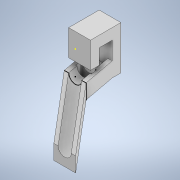
# Autodesk Inventor part: entry_ramp
Saved by Autodesk Inventor 2021 (Build 250183000, 183)
## iProperties
Created: 2021-04-02
Part Number: entry_ramp
Material: Generic
Document SubType Name: Modeling
Designer: Jawal
Density: 1 g/cm^3
Appearance: Default
Author: Jawal
Autodesk Inventor part; units mm, degrees
note: some values were not read from the file. Chosen so that the rebuilt part matches the saved one: direction of "Emboss1".
sketch "Sketch1" plane through (0, 0, 0) normal (0, 0, 1) x (1, 0, 0)
  line L0 (-12.5, 12.5) -> (12.5, 12.5)
  line L1 (12.5, 12.5) -> (12.5, -37.5)
  line L2 (12.5, -37.5) -> (-12.5, -37.5)
  line L3 (-12.5, -37.5) -> (-12.5, 12.5)
  point P0 (0, 0)
  dimension "d0" = 25
  dimension "d1" = 50
  dimension "d2" = 12.5
  dimension "d3" = 12.5
  constraints: 8 end point, 2 parallel, 1 horizontal, 1 perpendicular
  measures "d0" distance of L0.start L0.end
  measures "d1" distance of L0.end L1.end
  measures "d2" distance from line of L1 point (0, 0)
  measures "d3" distance from line of point (0, 0) L0
sketch "Sketch1 outline for Extrusion1" plane through (0, 0, 0) normal (0, 0, 1) x (1, 0, 0)
  line L0 (-12.5, 12.5) -> (-12.5, -37.5)
  line L1 (12.5, 12.5) -> (-12.5, 12.5)
  line L2 (12.5, -37.5) -> (12.5, 12.5)
  line L3 (-12.5, -37.5) -> (12.5, -37.5)
extrude "Extrusion1" add sketch "Sketch1 outline for Extrusion1" along normal blind 10
sketch "Sketch2" plane through (0, 0, 0) normal (0, 0, -1) x (-1, 0, 0)
  circle A0 centre (0, -33) radius 1.5
  circle A1 centre (0, 0) radius 7.5
  dimension "d7" = 3
  dimension "d8" = 33
  dimension "d17" = 15
  constraints: 2 centre point, 1 coincident
  measures "d7" diameter of A0
  measures "d8" distance of A0.centre point (0, 0)
  measures "d17" diameter of A1
sketch "Sketch2 outline for Extrusion2" plane through (0, 0, 0) normal (0, 0, -1) x (-1, 0, 0)
  circle A0 centre (0, -33) radius 1.5
extrude "Extrusion2" add sketch "Sketch2 outline for Extrusion2" along normal blind 6
sketch "Sketch3" plane through (0, 0, 10) normal (0, 0, 1) x (1, 0, 0)
  arc A0 (7.5, 0) -> (-7.5, 0) centre (0, 0) ccw
  line L0 (-7.5, 0) -> (-12.5, 0)
  line L1 (-12.5, 12.5) -> (-12.5, -37.5) projected
  line L2 (-12.5, 0) -> (-12.5, 12.5)
  line L3 (12.5, 12.5) -> (-12.5, 12.5) projected
  line L4 (12.5, 12.5) -> (12.5, 0)
  line L5 (12.5, -37.5) -> (12.5, 12.5) projected
  line L6 (7.5, 0) -> (12.5, 0)
  dimension "d11" = 15
  constraints: 8 end point, 2 point on circle, 2 point on line, 1 centre point, 1 coincident, 1 collinear, 1 horizontal, 1 perpendicular
  measures "d11" diameter of A0
sketch "Sketch3 outline for Extrusion3" plane through (0, 0, 10) normal (0, 0, 1) x (1, 0, 0)
  arc A0 (-7.5, 0) -> (7.5, 0) centre (0, 0) cw
  line L0 (-12.5, 0) -> (-7.5, 0)
  line L1 (-12.5, 12.5) -> (-12.5, 0)
  line L2 (12.5, 12.5) -> (-12.5, 12.5)
  line L3 (12.5, 0) -> (12.5, 12.5)
  line L4 (7.5, 0) -> (12.5, 0)
extrude "Extrusion3" add sketch "Sketch3 outline for Extrusion3" along normal blind 15
sketch "Sketch4" plane through (0, 0, 25) normal (0, 0, 1) x (1, 0, 0)
  line L0 (-12.5, 12.5) -> (-12.5, 0) projected
  line L1 (-12.5, 12.5) -> (12.5, 12.5)
  line L2 (12.5, 12.5) -> (12.5, -17.5)
  line L3 (12.5, -17.5) -> (-12.5, -17.5)
  line L4 (-12.5, -17.5) -> (-12.5, 12.5)
  point P0 (0, 0)
  dimension "d14" = 25
  dimension "d21" = 30
  constraints: 8 end point, 2 parallel, 1 horizontal, 1 perpendicular
  measures "d14" distance of L2.end L3.end
  measures "d21" distance of L1.end L2.end
sketch "Sketch4 outline for Extrusion4" plane through (0, 0, 25) normal (0, 0, 1) x (1, 0, 0)
  line L0 (-12.5, -17.5) -> (12.5, -17.5)
  line L1 (-12.5, 0) -> (-12.5, -17.5)
  line L2 (-12.5, 12.5) -> (-12.5, 0)
  line L3 (12.5, 12.5) -> (-12.5, 12.5)
  line L4 (12.5, -17.5) -> (12.5, 12.5)
extrude "Extrusion4" add sketch "Sketch4 outline for Extrusion4" along normal blind 10
sketch "Sketch5" plane through (0, 0, 0) normal (0, 0, -1) x (-1, 0, 0)
  circle A0 centre (0, 0) radius 7.5
  dimension "d18" = 15
  constraints: 1 centre point, 1 coincident
  measures "d18" diameter of A0
sketch "Sketch5 outline for Extrusion5" plane through (0, 0, 0) normal (0, 0, -1) x (-1, 0, 0)
  circle A0 centre (0, 0) radius 7.5
extrude "Extrusion5" cut sketch "Sketch5 outline for Extrusion5" against normal blind 10
sketch "Sketch6" plane through (0, 0, 10) normal (0, 0, 1) x (1, 0, 0)
  line L0 (-12.5, -20.5) -> (-12.5, -37.5)
  line L1 (-12.5, -37.5) -> (12.5, -37.5) projected
  line L2 (-12.5, -37.5) -> (12.5, -37.5)
  line L3 (12.5, -37.5) -> (12.5, -20.5)
  line L4 (12.5, -37.5) -> (12.5, 0) projected
  arc A0 (-7.5, -20.5) -> (7.5, -20.5) centre (0, -20.5) ccw
  line L5 (-12.5, -20.5) -> (-7.5, -20.5)
  line L6 (7.5, -20.5) -> (12.5, -20.5)
  line L7 (-12.5, 0) -> (-12.5, -37.5) projected
  line L8 (-12.5, -29) -> (12.5, -29)
  point P0 (0, 0)
  dimension "d22" = 15
  dimension "d23" = 17
  dimension "d24" = 17
  constraints: 12 end point, 3 point on line, 2 horizontal, 2 point on circle, 1 centre point, 1 collinear, 1 perpendicular
  measures "d22" diameter of A0
  measures "d23" distance of L1.end L3.end
  measures "d24" distance of L0.start L0.end
ref_plane "Work Plane1" through (0, -37.5, 0) normal (-1, 0, 0) x (0, 0, 1)
sketch "Sketch8" plane through (0, -37.5, 0) normal (-1, 0, 0) x (0, 0, 1)
  line L0 (10, 0) -> (10, 37.5)
  line L1 (10, 8.5) -> (40, 1.573954)
  line L2 (10, 8.5) -> (40.789123, 8.5) construction
  line L3 (0, 0) -> (10, 0)
  point P0 (0, 37.5)
  dimension "d26" = 13
  dimension "d27" = 8.5
  dimension "d32" = 30
  constraints: 4 end point, 1 equal length, 1 horizontal, 1 point on line
  measures "d26" angle of L1 L2
  measures "d27" distance between parallel lines of L3 L2
  measures "d32" distance from line of L1.end L0
sketch "Sketch6 outline for Sweep1" plane through (0, 0, 10) normal (0, 0, 1) x (1, 0, 0)
  arc A0 (7.5, -20.5) -> (-7.5, -20.5) centre (0, -20.5) cw
  line L0 (12.5, -20.5) -> (7.5, -20.5)
  line L1 (12.5, -37.5) -> (12.5, -20.5)
  line L2 (-12.5, -37.5) -> (12.5, -37.5)
  line L3 (-12.5, -20.5) -> (-12.5, -37.5)
  line L4 (-7.5, -20.5) -> (-12.5, -20.5)
sweep "Sweep1" add profiles "Sketch6 outline for Sweep1" path "Sketch8" path curves L1
thread "Thread1"
sketch "Sketch9" plane through (-12.5, -44.426046, 40) normal (0, 0, 1) x (1, 0, 0)
  point P0 (12.5, 44.426046)
sketch "Sketch10" plane through (-12.5, -44.426046, 40) normal (0, 0, 1) x (1, 0, 0)
  point P0 (12.5, 44.426046)
ref_plane "Work Plane2" through (12.5, -44.426046, 40) normal (0, -1, 0) x (1, 0, 0)
sketch "Sketch12" plane through (12.5, -44.426046, 40) normal (0, -1, 0) x (1, 0, 0)
  line L0 (-3.5, -15.5) -> (-21.5, -15.5)
  line L1 (-21.5, -15.5) -> (-21.5, -9.5)
  line L2 (-21.5, -9.5) -> (-3.5, -9.5)
  line L3 (-3.5, -9.5) -> (-3.5, -15.5)
  line L4 (0, -30) -> (0, 0) projected
  point P0 (-12.5, -40)
  dimension "d33" = 18
  dimension "d34" = 6
  dimension "d35" = 3.5
  dimension "d36" = 14.5
  constraints: 8 end point, 1 horizontal, 1 parallel, 1 perpendicular
  measures "d33" distance of L1.end L2.end
  measures "d34" distance of L0.end L1.end
  measures "d35" distance between parallel lines of L4 L3
  measures "d36" distance from line of L4.start L0
sketch "Sketch12 outline for Extrusion6" plane through (12.5, -44.426046, 40) normal (0, -1, 0) x (1, 0, 0)
  line L0 (-3.5, -15.5) -> (-3.5, -9.5)
  line L1 (-21.5, -15.5) -> (-3.5, -15.5)
  line L2 (-21.5, -9.5) -> (-21.5, -15.5)
  line L3 (-3.5, -9.5) -> (-21.5, -9.5)
extrude "Extrusion6" cut sketch "Sketch12 outline for Extrusion6" against normal blind 25
sketch "Sketch13" plane through (-12.5, -44.426046, 40) normal (0, 0, 1) x (1, 0, 0)
  line L0 (5, 17) -> (0, 17) projected
  line L1 (5, 17) -> (0, 17)
  line L2 (0, 17) -> (0, 0) projected
  line L3 (0, 17) -> (0, 0)
  line L4 (0, 0) -> (25, 0) projected
  line L5 (0, 0) -> (25, 0)
  line L6 (25, 0) -> (25, 17) projected
  line L7 (25, 0) -> (25, 17)
  arc A0 (5, 17) -> (20, 17) centre (12.5, 17) ccw projected
  line L8 (25, 17) -> (20, 17)
  arc A1 (5, 17) -> (20, 17) centre (12.5, 17) ccw
  point P0 (12.5, 44.426046)
  constraints: 10 end point, 2 collinear, 2 perpendicular, 2 point on circle, 1 centre point, 1 concentric, 1 horizontal
ref_plane "Work Plane3" through (-12.5, -44.426046, 80) normal (0, 0, 1) x (1, 0, 0)
sketch "Sketch14" plane through (-12.5, -44.426046, 80) normal (0, 0, 1) x (1, 0, 0)
  line L0 (28, -21.574) -> (28, -38.574)
  line L1 (28, -38.574) -> (53, -38.574)
  line L2 (53, -38.574) -> (53, -21.574)
  line L3 (53, -21.574) -> (48, -21.574)
  line L4 (28, -21.574) -> (33, -21.574)
  arc A0 (33, -21.574) -> (48, -21.574) centre (40.5, -21.574) ccw
  line L5 (5, 17) -> (0, 17) projected
  point P0 (12.5, 44.426046)
  dimension "d40" = 17
  dimension "d41" = 25
  dimension "d42" = 5
  dimension "d43" = 5
  dimension "d45" = 15
  dimension "d46" = 38.574
  dimension "d47" = 28
  constraints: 10 end point, 3 perpendicular, 2 point on circle, 1 centre point, 1 horizontal, 1 vertical
  measures "d40" distance of L0.start L0.end
  measures "d41" distance of L0.end L1.end
  measures "d42" distance of L2.end L3.end
  measures "d43" distance of L0.start L4.end
  measures "d45" diameter of A0
  measures "d46" distance between parallel lines of L4 L5
  measures "d47" horizontal distance of L0.start L5.end
sketch "Sketch14 outline for Loft1" plane through (-12.5, -44.426046, 80) normal (0, 0, 1) x (1, 0, 0)
  line L0 (33, -21.574) -> (28, -21.574)
  arc A0 (48, -21.574) -> (33, -21.574) centre (40.5, -21.574) cw
  line L1 (53, -21.574) -> (48, -21.574)
  line L2 (53, -38.574) -> (53, -21.574)
  line L3 (28, -38.574) -> (53, -38.574)
  line L4 (28, -21.574) -> (28, -38.574)
loft "Loft1" add profiles "Sketch14 outline for Loft1" section 1 edges at (-10, -27.426046, 40) (-12.5, -35.926046, 40) (0, -44.426046, 40) (12.5, -35.926046, 40) (10, -27.426046, 40) (0, -34.926046, 40)
sketch "Sketch15" plane through (-12.5, -37.5, 0) normal (-1, 0, 0) x (0, 0, 1)
  line L0 (6.091781, 45.785955) -> (39.829507, 45.785955) construction
  line L1 (39.829507, 45.785955) -> (39.829507, 34.540045) construction
  line L2 (39.829507, 34.540045) -> (6.091781, 34.540045) construction
  line L3 (6.091781, 34.540045) -> (6.091781, 45.785955) construction
  line L4 (6.400533, 42.737955) -> (6.400533, 45.785955)
  line L5 (6.400533, 45.785955) -> (8.307386, 45.785955)
  line L6 (8.307386, 45.785955) -> (8.307386, 45.425332)
  line L7 (8.307386, 45.425332) -> (6.805616, 45.425332)
  line L8 (6.805616, 45.425332) -> (6.805616, 44.590467)
  line L9 (6.805616, 44.590467) -> (8.206115, 44.590467)
  line L10 (8.206115, 44.590467) -> (8.206115, 44.229844)
  line L11 (8.206115, 44.229844) -> (6.805616, 44.229844)
  line L12 (6.805616, 44.229844) -> (6.805616, 43.098577)
  line L13 (6.805616, 43.098577) -> (8.307386, 43.098577)
  line L14 (8.307386, 43.098577) -> (8.307386, 42.737955)
  line L15 (8.307386, 42.737955) -> (6.400533, 42.737955)
  line L16 (10.51805, 42.737955) -> (10.132728, 42.737955)
  line L17 (10.132728, 42.737955) -> (10.132728, 44.042123)
  spline S0 degree 2 poles (10.132728, 44.042123) (10.132728, 44.200204) (10.103087, 44.471906) (10.058627, 44.553417) knots 0 0 0 1 2 2 2
  spline S1 degree 2 poles (10.058627, 44.553417) (10.011697, 44.639867) (9.843736, 44.723848) (9.700475, 44.723848) knots 0 0 0 1 2 2 2
  spline S2 degree 2 poles (9.700475, 44.723848) (9.557214, 44.723848) (9.253402, 44.570707) (9.107671, 44.447206) knots 0 0 0 1 2 2 2
  line L18 (9.107671, 44.447206) -> (9.107671, 42.737955)
  line L19 (9.107671, 42.737955) -> (8.722348, 42.737955)
  line L20 (8.722348, 42.737955) -> (8.722348, 45.02519)
  line L21 (8.722348, 45.02519) -> (9.107671, 45.02519)
  line L22 (9.107671, 45.02519) -> (9.107671, 44.770778)
  spline S3 degree 2 poles (9.107671, 44.770778) (9.280572, 44.926389) (9.614024, 45.08941) (9.801745, 45.08941) knots 0 0 0 1 2 2 2
  spline S4 degree 2 poles (9.801745, 45.08941) (10.137668, 45.08941) (10.51805, 44.644807) (10.51805, 44.222434) knots 0 0 0 1 2 2 2
  line L23 (10.51805, 44.222434) -> (10.51805, 42.737955)
  spline S5 degree 2 poles (11.750588, 42.693494) (11.436896, 42.693494) (11.083684, 43.051647) (11.083684, 43.439439) knots 0 0 0 1 2 2 2
  line L24 (11.083684, 43.439439) -> (11.083684, 44.706558)
  line L25 (11.083684, 44.706558) -> (10.824332, 44.706558)
  line L26 (10.824332, 44.706558) -> (10.824332, 45.02519)
  line L27 (10.824332, 45.02519) -> (11.083684, 45.02519)
  line L28 (11.083684, 45.02519) -> (11.083684, 45.682214)
  line L29 (11.083684, 45.682214) -> (11.469006, 45.682214)
  line L30 (11.469006, 45.682214) -> (11.469006, 45.02519)
  line L31 (11.469006, 45.02519) -> (12.177901, 45.02519)
  line L32 (12.177901, 45.02519) -> (12.177901, 44.706558)
  line L33 (12.177901, 44.706558) -> (11.469006, 44.706558)
  line L34 (11.469006, 44.706558) -> (11.469006, 43.61728)
  spline S6 degree 2 poles (11.469006, 43.61728) (11.469006, 43.444379) (11.481356, 43.254188) (11.523347, 43.172678) knots 0 0 0 1 2 2 2
  spline S7 degree 2 poles (11.523347, 43.172678) (11.557927, 43.101047) (11.713538, 43.029417) (11.846919, 43.029417) knots 0 0 0 1 2 2 2
  spline S8 degree 2 poles (11.846919, 43.029417) (11.940779, 43.029417) (12.116151, 43.086227) (12.155671, 43.103517) knots 0 0 0 1 2 2 2
  line L35 (12.155671, 43.103517) -> (12.177901, 43.103517)
  line L36 (12.177901, 43.103517) -> (12.177901, 42.757715)
  spline S9 degree 2 poles (12.177901, 42.757715) (12.06922, 42.728075) (11.846919, 42.693494) (11.750588, 42.693494) knots 0 0 0 1 2 2 2
  line L37 (13.674731, 44.612697) -> (13.654971, 44.612697)
  spline S10 degree 2 poles (13.654971, 44.612697) (13.61051, 44.625047) (13.51418, 44.629987) (13.447489, 44.629987) knots 0 0 0 1 2 2 2
  spline S11 degree 2 poles (13.447489, 44.629987) (13.291878, 44.629987) (12.985596, 44.494136) (12.847275, 44.360755) knots 0 0 0 1 2 2 2
  line L38 (12.847275, 44.360755) -> (12.847275, 42.737955)
  line L39 (12.847275, 42.737955) -> (12.461953, 42.737955)
  line L40 (12.461953, 42.737955) -> (12.461953, 45.02519)
  line L41 (12.461953, 45.02519) -> (12.847275, 45.02519)
  line L42 (12.847275, 45.02519) -> (12.847275, 44.684327)
  spline S12 degree 2 poles (12.847275, 44.684327) (13.057227, 44.872049) (13.370919, 45.02519) (13.51912, 45.02519) knots 0 0 0 1 2 2 2
  spline S13 degree 2 poles (13.51912, 45.02519) (13.5784, 45.02519) (13.637681, 45.02025) (13.674731, 45.01284) knots 0 0 0 1 2 2 2
  line L43 (13.674731, 45.01284) -> (13.674731, 44.612697)
  line L44 (15.769305, 45.02519) -> (14.539237, 41.895679)
  line L45 (14.539237, 41.895679) -> (14.126744, 41.895679)
  line L46 (14.126744, 41.895679) -> (14.536767, 42.849105)
  line L47 (14.536767, 42.849105) -> (13.706841, 45.02519)
  line L48 (13.706841, 45.02519) -> (14.121804, 45.02519)
  line L49 (14.121804, 45.02519) -> (14.746718, 43.330759)
  line L50 (14.746718, 43.330759) -> (15.369162, 45.02519)
  line L51 (15.369162, 45.02519) -> (15.769305, 45.02519)
  line L52 (19.758381, 42.737955) -> (19.232267, 42.737955)
  line L53 (19.232267, 42.737955) -> (18.268961, 43.950733)
  line L54 (18.268961, 43.950733) -> (17.804598, 43.950733)
  line L55 (17.804598, 43.950733) -> (17.804598, 42.737955)
  line L56 (17.804598, 42.737955) -> (17.399515, 42.737955)
  line L57 (17.399515, 42.737955) -> (17.399515, 45.785955)
  line L58 (17.399515, 45.785955) -> (18.184981, 45.785955)
  spline S14 degree 2 poles (18.184981, 45.785955) (18.446802, 45.785955) (18.800015, 45.729144) (18.960566, 45.625404) knots 0 0 0 1 2 2 2
  spline S15 degree 2 poles (18.960566, 45.625404) (19.121117, 45.521663) (19.306368, 45.198091) (19.306368, 44.958499) knots 0 0 0 1 2 2 2
  spline S16 degree 2 poles (19.306368, 44.958499) (19.306368, 44.625047) (18.965506, 44.173034) (18.674044, 44.064353) knots 0 0 0 1 2 2 2
  line L59 (18.674044, 44.064353) -> (19.758381, 42.737955)
  spline S17 degree 2 poles (18.883995, 44.926389) (18.883995, 45.05977) (18.790135, 45.264781) (18.691334, 45.331472) knots 0 0 0 1 2 2 2
  spline S18 degree 2 poles (18.691334, 45.331472) (18.604883, 45.388282) (18.375172, 45.435212) (18.207211, 45.435212) knots 0 0 0 1 2 2 2
  line L60 (18.207211, 45.435212) -> (17.804598, 45.435212)
  line L61 (17.804598, 45.435212) -> (17.804598, 44.289125)
  line L62 (17.804598, 44.289125) -> (18.16028, 44.289125)
  spline S19 degree 2 poles (18.16028, 44.289125) (18.335652, 44.289125) (18.614763, 44.350875) (18.711094, 44.447206) knots 0 0 0 1 2 2 2
  spline S20 degree 2 poles (18.711094, 44.447206) (18.800015, 44.531186) (18.883995, 44.768308) (18.883995, 44.926389) knots 0 0 0 1 2 2 2
  spline S21 degree 2 poles (21.245331, 42.980016) (21.1984, 42.945436) (21.040319, 42.821935) (20.966219, 42.784885) knots 0 0 0 1 2 2 2
  spline S22 degree 2 poles (20.966219, 42.784885) (20.864948, 42.730545) (20.674757, 42.673734) (20.501856, 42.673734) knots 0 0 0 1 2 2 2
  spline S23 degree 2 poles (20.501856, 42.673734) (20.361065, 42.673734) (20.106653, 42.779945) (20.010323, 42.876276) knots 0 0 0 1 2 2 2
  spline S24 degree 2 poles (20.010323, 42.876276) (19.918932, 42.970136) (19.807781, 43.246778) (19.807781, 43.399919) knots 0 0 0 1 2 2 2
  spline S25 degree 2 poles (19.807781, 43.399919) (19.807781, 43.637041) (20.007853, 43.972963) (20.225214, 44.069293) knots 0 0 0 1 2 2 2
  spline S26 degree 2 poles (20.225214, 44.069293) (20.417875, 44.158214) (20.941519, 44.224904) (21.245331, 44.242195) knots 0 0 0 1 2 2 2
  line L63 (21.245331, 44.242195) -> (21.245331, 44.316295)
  spline S27 degree 2 poles (21.245331, 44.316295) (21.245331, 44.449676) (21.16382, 44.615167) (21.08972, 44.662097) knots 0 0 0 1 2 2 2
  spline S28 degree 2 poles (21.08972, 44.662097) (21.015619, 44.709028) (20.803198, 44.738668) (20.689577, 44.738668) knots 0 0 0 1 2 2 2
  spline S29 degree 2 poles (20.689577, 44.738668) (20.556196, 44.738668) (20.195574, 44.659627) (20.015263, 44.583057) knots 0 0 0 1 2 2 2
  line L64 (20.015263, 44.583057) -> (19.993032, 44.583057)
  line L65 (19.993032, 44.583057) -> (19.993032, 44.975789)
  spline S30 degree 2 poles (19.993032, 44.975789) (20.099243, 45.00543) (20.496916, 45.07953) (20.692047, 45.07953) knots 0 0 0 1 2 2 2
  spline S31 degree 2 poles (20.692047, 45.07953) (20.929169, 45.07953) (21.252741, 45.00543) (21.381182, 44.909099) knots 0 0 0 1 2 2 2
  spline S32 degree 2 poles (21.381182, 44.909099) (21.507152, 44.815238) (21.630653, 44.516366) (21.630653, 44.301475) knots 0 0 0 1 2 2 2
  line L66 (21.630653, 44.301475) -> (21.630653, 42.737955)
  line L67 (21.630653, 42.737955) -> (21.245331, 42.737955)
  line L68 (21.245331, 42.737955) -> (21.245331, 42.980016)
  line L69 (21.245331, 43.301118) -> (21.245331, 43.935913)
  spline S33 degree 2 poles (21.245331, 43.935913) (21.10701, 43.923562) (20.689577, 43.881572) (20.558666, 43.842052) knots 0 0 0 1 2 2 2
  spline S34 degree 2 poles (20.558666, 43.842052) (20.405525, 43.795122) (20.205454, 43.59999) (20.205454, 43.427089) knots 0 0 0 1 2 2 2
  spline S35 degree 2 poles (20.205454, 43.427089) (20.205454, 43.229488) (20.427755, 43.029417) (20.640177, 43.029417) knots 0 0 0 1 2 2 2
  spline S36 degree 2 poles (20.640177, 43.029417) (20.820488, 43.029417) (21.11689, 43.185028) (21.245331, 43.301118) knots 0 0 0 1 2 2 2
  line L70 (24.765104, 42.737955) -> (24.765104, 44.061883)
  spline S37 degree 2 poles (24.765104, 44.061883) (24.765104, 44.219964) (24.740404, 44.489196) (24.700883, 44.563297) knots 0 0 0 1 2 2 2
  spline S38 degree 2 poles (24.700883, 44.563297) (24.661363, 44.644807) (24.510692, 44.723848) (24.379781, 44.723848) knots 0 0 0 1 2 2 2
  spline S39 degree 2 poles (24.379781, 44.723848) (24.26122, 44.723848) (23.989519, 44.578117) (23.846258, 44.439796) knots 0 0 0 1 2 2 2
  spline S40 degree 2 poles (23.846258, 44.439796) (23.848728, 44.405216) (23.853668, 44.308885) (23.853668, 44.244665) knots 0 0 0 1 2 2 2
  line L71 (23.853668, 44.244665) -> (23.853668, 42.737955)
  line L72 (23.853668, 42.737955) -> (23.468345, 42.737955)
  line L73 (23.468345, 42.737955) -> (23.468345, 44.061883)
  spline S41 degree 2 poles (23.468345, 44.061883) (23.468345, 44.219964) (23.443645, 44.489196) (23.404125, 44.563297) knots 0 0 0 1 2 2 2
  spline S42 degree 2 poles (23.404125, 44.563297) (23.364605, 44.644807) (23.213934, 44.723848) (23.083023, 44.723848) knots 0 0 0 1 2 2 2
  spline S43 degree 2 poles (23.083023, 44.723848) (22.959522, 44.723848) (22.68535, 44.568237) (22.556909, 44.447206) knots 0 0 0 1 2 2 2
  line L74 (22.556909, 44.447206) -> (22.556909, 42.737955)
  line L75 (22.556909, 42.737955) -> (22.171587, 42.737955)
  line L76 (22.171587, 42.737955) -> (22.171587, 45.02519)
  line L77 (22.171587, 45.02519) -> (22.556909, 45.02519)
  line L78 (22.556909, 45.02519) -> (22.556909, 44.773248)
  spline S44 degree 2 poles (22.556909, 44.773248) (22.70758, 44.923919) (23.003982, 45.08941) (23.181823, 45.08941) knots 0 0 0 1 2 2 2
  spline S45 degree 2 poles (23.181823, 45.08941) (23.384365, 45.08941) (23.698057, 44.904159) (23.779567, 44.694208) knots 0 0 0 1 2 2 2
  spline S46 degree 2 poles (23.779567, 44.694208) (23.954938, 44.889339) (24.285921, 45.08941) (24.478582, 45.08941) knots 0 0 0 1 2 2 2
  spline S47 degree 2 poles (24.478582, 45.08941) (24.626783, 45.08941) (24.868844, 44.99802) (24.957765, 44.894279) knots 0 0 0 1 2 2 2
  spline S48 degree 2 poles (24.957765, 44.894279) (25.049156, 44.790538) (25.150426, 44.479316) (25.150426, 44.244665) knots 0 0 0 1 2 2 2
  line L79 (25.150426, 44.244665) -> (25.150426, 42.737955)
  line L80 (25.150426, 42.737955) -> (24.765104, 42.737955)
  spline S49 degree 2 poles (27.608092, 43.943323) (27.608092, 43.370279) (27.062219, 42.693494) (26.644786, 42.693494) knots 0 0 0 1 2 2 2
  spline S50 degree 2 poles (26.644786, 42.693494) (26.474355, 42.693494) (26.212533, 42.772535) (26.076682, 42.854045) knots 0 0 0 1 2 2 2
  line L81 (26.076682, 42.854045) -> (26.076682, 41.895679)
  line L82 (26.076682, 41.895679) -> (25.69136, 41.895679)
  line L83 (25.69136, 41.895679) -> (25.69136, 45.02519)
  line L84 (25.69136, 45.02519) -> (26.076682, 45.02519)
  line L85 (26.076682, 45.02519) -> (26.076682, 44.785598)
  spline S51 degree 2 poles (26.076682, 44.785598) (26.219943, 44.916509) (26.570686, 45.08941) (26.775697, 45.08941) knots 0 0 0 1 2 2 2
  spline S52 degree 2 poles (26.775697, 45.08941) (27.16843, 45.08941) (27.608092, 44.466966) (27.608092, 43.943323) knots 0 0 0 1 2 2 2
  spline S53 degree 2 poles (27.21042, 43.898862) (27.21042, 44.291595) (26.960948, 44.723848) (26.681836, 44.723848) knots 0 0 0 1 2 2 2
  spline S54 degree 2 poles (26.681836, 44.723848) (26.518815, 44.723848) (26.212533, 44.578117) (26.076682, 44.464496) knots 0 0 0 1 2 2 2
  line L86 (26.076682, 44.464496) -> (26.076682, 43.165267)
  spline S55 degree 2 poles (26.076682, 43.165267) (26.227353, 43.093637) (26.442245, 43.039297) (26.580566, 43.039297) knots 0 0 0 1 2 2 2
  spline S56 degree 2 poles (26.580566, 43.039297) (26.879438, 43.039297) (27.21042, 43.47896) (27.21042, 43.898862) knots 0 0 0 1 2 2 2
  point P0 (0, 37.5)
  constraints: 2 other
sketch "Sketch15 outline for Emboss1" plane through (-12.5, -37.5, 0) normal (-1, 0, 0) x (0, 0, 1)
  line L0 (6.400533, 42.737955) -> (6.400533, 45.785955)
  line L1 (6.400533, 45.785955) -> (8.307386, 45.785955)
  line L2 (8.307386, 45.785955) -> (8.307386, 45.425332)
  line L3 (8.307386, 45.425332) -> (6.805616, 45.425332)
  line L4 (6.805616, 45.425332) -> (6.805616, 44.590467)
  line L5 (6.805616, 44.590467) -> (8.206115, 44.590467)
  line L6 (8.206115, 44.590467) -> (8.206115, 44.229844)
  line L7 (8.206115, 44.229844) -> (6.805616, 44.229844)
  line L8 (6.805616, 44.229844) -> (6.805616, 43.098577)
  line L9 (6.805616, 43.098577) -> (8.307386, 43.098577)
  line L10 (8.307386, 43.098577) -> (8.307386, 42.737955)
  line L11 (8.307386, 42.737955) -> (6.400533, 42.737955)
  line L12 (10.51805, 42.737955) -> (10.132728, 42.737955)
  line L13 (10.132728, 42.737955) -> (10.132728, 44.042123)
  spline S0 degree 2 poles (10.132728, 44.042123) (10.132728, 44.200204) (10.103087, 44.471906) (10.058627, 44.553417) knots 0 0 0 0.5 1 1 1
  spline S1 degree 2 poles (10.058627, 44.553417) (10.011697, 44.639867) (9.843736, 44.723848) (9.700475, 44.723848) knots 0 0 0 0.5 1 1 1
  spline S2 degree 2 poles (9.700475, 44.723848) (9.557214, 44.723848) (9.253402, 44.570707) (9.107671, 44.447206) knots 0 0 0 0.5 1 1 1
  line L14 (9.107671, 44.447206) -> (9.107671, 42.737955)
  line L15 (9.107671, 42.737955) -> (8.722348, 42.737955)
  line L16 (8.722348, 42.737955) -> (8.722348, 45.02519)
  line L17 (8.722348, 45.02519) -> (9.107671, 45.02519)
  line L18 (9.107671, 45.02519) -> (9.107671, 44.770778)
  spline S3 degree 2 poles (9.107671, 44.770778) (9.280572, 44.926389) (9.614024, 45.08941) (9.801745, 45.08941) knots 0 0 0 0.5 1 1 1
  spline S4 degree 2 poles (9.801745, 45.08941) (10.137668, 45.08941) (10.51805, 44.644807) (10.51805, 44.222434) knots 0 0 0 0.5 1 1 1
  line L19 (10.51805, 44.222434) -> (10.51805, 42.737955)
  spline S5 degree 2 poles (11.750588, 42.693494) (11.436896, 42.693494) (11.083684, 43.051647) (11.083684, 43.439439) knots 0 0 0 0.5 1 1 1
  line L20 (11.083684, 43.439439) -> (11.083684, 44.706558)
  line L21 (11.083684, 44.706558) -> (10.824332, 44.706558)
  line L22 (10.824332, 44.706558) -> (10.824332, 45.02519)
  line L23 (10.824332, 45.02519) -> (11.083684, 45.02519)
  line L24 (11.083684, 45.02519) -> (11.083684, 45.682214)
  line L25 (11.083684, 45.682214) -> (11.469006, 45.682214)
  line L26 (11.469006, 45.682214) -> (11.469006, 45.02519)
  line L27 (11.469006, 45.02519) -> (12.177901, 45.02519)
  line L28 (12.177901, 45.02519) -> (12.177901, 44.706558)
  line L29 (12.177901, 44.706558) -> (11.469006, 44.706558)
  line L30 (11.469006, 44.706558) -> (11.469006, 43.61728)
  spline S6 degree 2 poles (11.469006, 43.61728) (11.469006, 43.444379) (11.481356, 43.254188) (11.523347, 43.172678) knots 0 0 0 0.5 1 1 1
  spline S7 degree 2 poles (11.523347, 43.172678) (11.557927, 43.101047) (11.713538, 43.029417) (11.846919, 43.029417) knots 0 0 0 0.5 1 1 1
  spline S8 degree 2 poles (11.846919, 43.029417) (11.940779, 43.029417) (12.116151, 43.086227) (12.155671, 43.103517) knots 0 0 0 0.5 1 1 1
  line L31 (12.155671, 43.103517) -> (12.177901, 43.103517)
  line L32 (12.177901, 43.103517) -> (12.177901, 42.757715)
  spline S9 degree 2 poles (12.177901, 42.757715) (12.06922, 42.728075) (11.846919, 42.693494) (11.750588, 42.693494) knots 0 0 0 0.5 1 1 1
  line L33 (13.674731, 44.612697) -> (13.654971, 44.612697)
  spline S10 degree 2 poles (13.654971, 44.612697) (13.61051, 44.625047) (13.51418, 44.629987) (13.447489, 44.629987) knots 0 0 0 0.5 1 1 1
  spline S11 degree 2 poles (13.447489, 44.629987) (13.291878, 44.629987) (12.985596, 44.494136) (12.847275, 44.360755) knots 0 0 0 0.5 1 1 1
  line L34 (12.847275, 44.360755) -> (12.847275, 42.737955)
  line L35 (12.847275, 42.737955) -> (12.461953, 42.737955)
  line L36 (12.461953, 42.737955) -> (12.461953, 45.02519)
  line L37 (12.461953, 45.02519) -> (12.847275, 45.02519)
  line L38 (12.847275, 45.02519) -> (12.847275, 44.684327)
  spline S12 degree 2 poles (12.847275, 44.684327) (13.057227, 44.872049) (13.370919, 45.02519) (13.51912, 45.02519) knots 0 0 0 0.5 1 1 1
  spline S13 degree 2 poles (13.51912, 45.02519) (13.5784, 45.02519) (13.637681, 45.02025) (13.674731, 45.01284) knots 0 0 0 0.5 1 1 1
  line L39 (13.674731, 45.01284) -> (13.674731, 44.612697)
  line L40 (15.769305, 45.02519) -> (14.539237, 41.895679)
  line L41 (14.539237, 41.895679) -> (14.126744, 41.895679)
  line L42 (14.126744, 41.895679) -> (14.536767, 42.849105)
  line L43 (14.536767, 42.849105) -> (13.706841, 45.02519)
  line L44 (13.706841, 45.02519) -> (14.121804, 45.02519)
  line L45 (14.121804, 45.02519) -> (14.746718, 43.330759)
  line L46 (14.746718, 43.330759) -> (15.369162, 45.02519)
  line L47 (15.369162, 45.02519) -> (15.769305, 45.02519)
  line L48 (19.758381, 42.737955) -> (19.232267, 42.737955)
  line L49 (18.674044, 44.064353) -> (19.758381, 42.737955)
  line L50 (19.232267, 42.737955) -> (18.268961, 43.950733)
  spline S14 degree 2 poles (19.306368, 44.958499) (19.306368, 44.625047) (18.965506, 44.173034) (18.674044, 44.064353) knots 0 0 0 0.5 1 1 1
  line L51 (18.268961, 43.950733) -> (17.804598, 43.950733)
  spline S15 degree 2 poles (18.960566, 45.625404) (19.121117, 45.521663) (19.306368, 45.198091) (19.306368, 44.958499) knots 0 0 0 0.5 1 1 1
  line L52 (17.804598, 43.950733) -> (17.804598, 42.737955)
  spline S16 degree 2 poles (18.184981, 45.785955) (18.446802, 45.785955) (18.800015, 45.729144) (18.960566, 45.625404) knots 0 0 0 0.5 1 1 1
  line L53 (17.804598, 42.737955) -> (17.399515, 42.737955)
  line L54 (17.399515, 45.785955) -> (18.184981, 45.785955)
  line L55 (17.399515, 42.737955) -> (17.399515, 45.785955)
  spline S17 degree 2 poles (18.711094, 44.447206) (18.800015, 44.531186) (18.883995, 44.768308) (18.883995, 44.926389) knots 0 0 0 0.5 1 1 1
  spline S18 degree 2 poles (18.883995, 44.926389) (18.883995, 45.05977) (18.790135, 45.264781) (18.691334, 45.331472) knots 0 0 0 0.5 1 1 1
  spline S19 degree 2 poles (18.691334, 45.331472) (18.604883, 45.388282) (18.375172, 45.435212) (18.207211, 45.435212) knots 0 0 0 0.5 1 1 1
  line L56 (18.207211, 45.435212) -> (17.804598, 45.435212)
  line L57 (17.804598, 45.435212) -> (17.804598, 44.289125)
  line L58 (17.804598, 44.289125) -> (18.16028, 44.289125)
  spline S20 degree 2 poles (18.16028, 44.289125) (18.335652, 44.289125) (18.614763, 44.350875) (18.711094, 44.447206) knots 0 0 0 0.5 1 1 1
  spline S21 degree 2 poles (21.245331, 42.980016) (21.1984, 42.945436) (21.040319, 42.821935) (20.966219, 42.784885) knots 0 0 0 0.5 1 1 1
  line L59 (21.245331, 42.737955) -> (21.245331, 42.980016)
  spline S22 degree 2 poles (20.966219, 42.784885) (20.864948, 42.730545) (20.674757, 42.673734) (20.501856, 42.673734) knots 0 0 0 0.5 1 1 1
  line L60 (21.630653, 42.737955) -> (21.245331, 42.737955)
  spline S23 degree 2 poles (20.501856, 42.673734) (20.361065, 42.673734) (20.106653, 42.779945) (20.010323, 42.876276) knots 0 0 0 0.5 1 1 1
  line L61 (21.630653, 44.301475) -> (21.630653, 42.737955)
  spline S24 degree 2 poles (20.010323, 42.876276) (19.918932, 42.970136) (19.807781, 43.246778) (19.807781, 43.399919) knots 0 0 0 0.5 1 1 1
  spline S25 degree 2 poles (21.381182, 44.909099) (21.507152, 44.815238) (21.630653, 44.516366) (21.630653, 44.301475) knots 0 0 0 0.5 1 1 1
  spline S26 degree 2 poles (19.807781, 43.399919) (19.807781, 43.637041) (20.007853, 43.972963) (20.225214, 44.069293) knots 0 0 0 0.5 1 1 1
  spline S27 degree 2 poles (20.692047, 45.07953) (20.929169, 45.07953) (21.252741, 45.00543) (21.381182, 44.909099) knots 0 0 0 0.5 1 1 1
  spline S28 degree 2 poles (20.225214, 44.069293) (20.417875, 44.158214) (20.941519, 44.224904) (21.245331, 44.242195) knots 0 0 0 0.5 1 1 1
  spline S29 degree 2 poles (19.993032, 44.975789) (20.099243, 45.00543) (20.496916, 45.07953) (20.692047, 45.07953) knots 0 0 0 0.5 1 1 1
  line L62 (21.245331, 44.242195) -> (21.245331, 44.316295)
  line L63 (19.993032, 44.583057) -> (19.993032, 44.975789)
  spline S30 degree 2 poles (21.245331, 44.316295) (21.245331, 44.449676) (21.16382, 44.615167) (21.08972, 44.662097) knots 0 0 0 0.5 1 1 1
  line L64 (20.015263, 44.583057) -> (19.993032, 44.583057)
  spline S31 degree 2 poles (21.08972, 44.662097) (21.015619, 44.709028) (20.803198, 44.738668) (20.689577, 44.738668) knots 0 0 0 0.5 1 1 1
  spline S32 degree 2 poles (20.689577, 44.738668) (20.556196, 44.738668) (20.195574, 44.659627) (20.015263, 44.583057) knots 0 0 0 0.5 1 1 1
  spline S33 degree 2 poles (20.640177, 43.029417) (20.820488, 43.029417) (21.11689, 43.185028) (21.245331, 43.301118) knots 0 0 0 0.5 1 1 1
  line L65 (21.245331, 43.301118) -> (21.245331, 43.935913)
  spline S34 degree 2 poles (21.245331, 43.935913) (21.10701, 43.923562) (20.689577, 43.881572) (20.558666, 43.842052) knots 0 0 0 0.5 1 1 1
  spline S35 degree 2 poles (20.558666, 43.842052) (20.405525, 43.795122) (20.205454, 43.59999) (20.205454, 43.427089) knots 0 0 0 0.5 1 1 1
  spline S36 degree 2 poles (20.205454, 43.427089) (20.205454, 43.229488) (20.427755, 43.029417) (20.640177, 43.029417) knots 0 0 0 0.5 1 1 1
  line L66 (24.765104, 42.737955) -> (24.765104, 44.061883)
  spline S37 degree 2 poles (24.765104, 44.061883) (24.765104, 44.219964) (24.740404, 44.489196) (24.700883, 44.563297) knots 0 0 0 0.5 1 1 1
  spline S38 degree 2 poles (24.700883, 44.563297) (24.661363, 44.644807) (24.510692, 44.723848) (24.379781, 44.723848) knots 0 0 0 0.5 1 1 1
  spline S39 degree 2 poles (24.379781, 44.723848) (24.26122, 44.723848) (23.989519, 44.578117) (23.846258, 44.439796) knots 0 0 0 0.5 1 1 1
  spline S40 degree 2 poles (23.846258, 44.439796) (23.848728, 44.405216) (23.853668, 44.308885) (23.853668, 44.244665) knots 0 0 0 0.5 1 1 1
  line L67 (23.853668, 44.244665) -> (23.853668, 42.737955)
  line L68 (23.853668, 42.737955) -> (23.468345, 42.737955)
  line L69 (23.468345, 42.737955) -> (23.468345, 44.061883)
  spline S41 degree 2 poles (23.468345, 44.061883) (23.468345, 44.219964) (23.443645, 44.489196) (23.404125, 44.563297) knots 0 0 0 0.5 1 1 1
  spline S42 degree 2 poles (23.404125, 44.563297) (23.364605, 44.644807) (23.213934, 44.723848) (23.083023, 44.723848) knots 0 0 0 0.5 1 1 1
  spline S43 degree 2 poles (23.083023, 44.723848) (22.959522, 44.723848) (22.68535, 44.568237) (22.556909, 44.447206) knots 0 0 0 0.5 1 1 1
  line L70 (22.556909, 44.447206) -> (22.556909, 42.737955)
  line L71 (22.556909, 42.737955) -> (22.171587, 42.737955)
  line L72 (22.171587, 42.737955) -> (22.171587, 45.02519)
  line L73 (22.171587, 45.02519) -> (22.556909, 45.02519)
  line L74 (22.556909, 45.02519) -> (22.556909, 44.773248)
  spline S44 degree 2 poles (22.556909, 44.773248) (22.70758, 44.923919) (23.003982, 45.08941) (23.181823, 45.08941) knots 0 0 0 0.5 1 1 1
  spline S45 degree 2 poles (23.181823, 45.08941) (23.384365, 45.08941) (23.698057, 44.904159) (23.779567, 44.694208) knots 0 0 0 0.5 1 1 1
  spline S46 degree 2 poles (23.779567, 44.694208) (23.954938, 44.889339) (24.285921, 45.08941) (24.478582, 45.08941) knots 0 0 0 0.5 1 1 1
  spline S47 degree 2 poles (24.478582, 45.08941) (24.626783, 45.08941) (24.868844, 44.99802) (24.957765, 44.894279) knots 0 0 0 0.5 1 1 1
  spline S48 degree 2 poles (24.957765, 44.894279) (25.049156, 44.790538) (25.150426, 44.479316) (25.150426, 44.244665) knots 0 0 0 0.5 1 1 1
  line L75 (25.150426, 44.244665) -> (25.150426, 42.737955)
  line L76 (25.150426, 42.737955) -> (24.765104, 42.737955)
  spline S49 degree 2 poles (27.608092, 43.943323) (27.608092, 43.370279) (27.062219, 42.693494) (26.644786, 42.693494) knots 0 0 0 0.5 1 1 1
  spline S50 degree 2 poles (26.775697, 45.08941) (27.16843, 45.08941) (27.608092, 44.466966) (27.608092, 43.943323) knots 0 0 0 0.5 1 1 1
  spline S51 degree 2 poles (26.644786, 42.693494) (26.474355, 42.693494) (26.212533, 42.772535) (26.076682, 42.854045) knots 0 0 0 0.5 1 1 1
  spline S52 degree 2 poles (26.076682, 44.785598) (26.219943, 44.916509) (26.570686, 45.08941) (26.775697, 45.08941) knots 0 0 0 0.5 1 1 1
  line L77 (26.076682, 42.854045) -> (26.076682, 41.895679)
  line L78 (26.076682, 45.02519) -> (26.076682, 44.785598)
  line L79 (26.076682, 41.895679) -> (25.69136, 41.895679)
  line L80 (25.69136, 45.02519) -> (26.076682, 45.02519)
  line L81 (25.69136, 41.895679) -> (25.69136, 45.02519)
  spline S53 degree 2 poles (26.580566, 43.039297) (26.879438, 43.039297) (27.21042, 43.47896) (27.21042, 43.898862) knots 0 0 0 0.5 1 1 1
  spline S54 degree 2 poles (27.21042, 43.898862) (27.21042, 44.291595) (26.960948, 44.723848) (26.681836, 44.723848) knots 0 0 0 0.5 1 1 1
  spline S55 degree 2 poles (26.681836, 44.723848) (26.518815, 44.723848) (26.212533, 44.578117) (26.076682, 44.464496) knots 0 0 0 0.5 1 1 1
  line L82 (26.076682, 44.464496) -> (26.076682, 43.165267)
  spline S56 degree 2 poles (26.076682, 43.165267) (26.227353, 43.093637) (26.442245, 43.039297) (26.580566, 43.039297) knots 0 0 0 0.5 1 1 1
emboss "Emboss1" sketch "Sketch15 outline for Emboss1" operation cut depth 1 direction (1, 0, 0)
equation "\"d2\" = 0.5 * d0"
equation "\"d24\" = d23"
body "Solid1"
